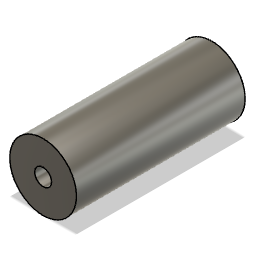
gasChargingCartridgePlug v9 (Autodesk Fusion 360 design; units mm, degrees)
Autodesk Fusion 360 part; units mm, degrees
note: some values were not read from the file. Chosen so that the rebuilt part matches the saved one: which face or edge a step refers to; a direction; where a thread starts; which pieces of a blend or face edit are solid.
sketch "Sketch3" plane through (0, 0, 0) normal (1, 0, 0) x (0, 0, -1)
  line L0 (0, 0) -> (-40, 0)
  line L1 (0, 0) -> (0, 7.9)
  line L2 (0, 7.9) -> (-40, 7.9)
  line L3 (-40, 7.9) -> (-40, 0)
  dimension "d23" = 7.9
  dimension "d24" = 40
  constraint coincident L0.start L1.start
  constraint horizontal L0
  constraint perpendicular L0 L1
  constraint perpendicular L1 L2
  constraint perpendicular L0 L3
  measures "d23" distance of L0.start L1.end
  measures "d24" distance of L0.start L0.end
revolve "Revolve1" add sketch "Sketch3" angle 360 about axis through (0, 0, 0) along (0, 0, 1) makes body 1
hole "Hole4" at (0, 0, 0) direction (0, 0, 1) diameter 4.234 depth 5 tip angle 118 bodies 1
thread "Thread3" "ISO Metric profile 5.0 M5x0.8 6H" major diameter 5.12 minor diameter 4.234 pitch 0.8 angle 60 modelled right hand crest width 0.2219 on face at (0.1055, 2.1144, 1.6667) crest through (0, 2.117, 5.6) on bodies 1
hole "Hole5" at (0, 0, 40) direction (0, 0, -1) diameter 4 depth 30 tip angle 118 bodies 1
sketch "Sketch4" plane through (0, 0, 0) normal (1, 0, 0) x (0, 0, -1)
  line L0 (-5, -11.7983) -> (-20, -11.7983)
  line L1 (-20, -11.7983) -> (-20, 8)
  line L2 (-20, 8) -> (-5, 8)
  line L3 (-5, 8) -> (-5, -11.7983)
  line L4 (0, -7.9) -> (0, 7.9)
  dimension "d32" = 15
  dimension "d33" = 5
  constraint horizontal L0
  constraint vertical L1
  constraint horizontal L2
  constraint vertical L3
  measures "d32" distance of L0.start L0.end
  measures "d33" distance of L3 L4
extrude "Extrude4" cut sketch "Sketch4" against normal blind 1 from surface at 8 bodies 1
hole "Hole6" at (7, 0, 12.5) direction (-1, 0, 0) diameter 3.332 depth 7 tip angle 118 bodies 1
thread "Thread4" "ISO Metric profile 4.0 M4x0.7 6H" thread offset 0 thread depth 10
copy_body "Körper->Berechn1" bodies 1 removing the originals makes body 2 in component "Component"
delete_face "Fläche löschen1" 1 faces at (5.0355, 1.666, 12.4996) on bodies 2 in component "Component"
delete_face "Fläche löschen2" 1 faces at (7, -1.2207, 10) on bodies 2 in component "Component"
ref_plane "Arbeitsebene2" through (0, -8, 0) normal (0, 1, 0) x (0, 0, 1)
sketch "Skizze5" plane through (0, -8, 0) normal (0, 1, 0) x (1, 0, 0)
  point P0 (0, -10)
  dimension "d41" = 10
  measures "d41" distance of origin P0
hole "Bohrung1" at (0, -8, 10) direction (0, 1, 0) diameter 1.623 depth 4 tip angle 118 bodies 2 in component "Component"
thread "Gewinde1" "ISO Metric profile 2.0 M2x0.4 6H" thread offset 0 thread depth 10 in component "Component"
component "Component" placed x (1, 0, 0) y (0, 1, 0) z (0, 0, 1) at (0, 0, 0)
equation "d23 = ( 15.8 / 2 ) * 1 mm"
